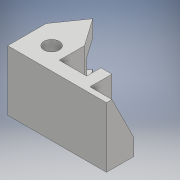
# Autodesk Inventor part: P4-10
Saved by Autodesk Inventor 2017 (Build 210142000, 142)
## iProperties
Created: 2017-03-01
Part Number: P4-10
Material: Generic
Document SubType Name: Modeling
Designer: Schaffel
Density: 1 g/cm^3
Appearance: Default
Author: Schaffel
Autodesk Inventor part; units mm, degrees
ref_plane "YZ Plane" through (0, 0, 0) normal (1, 0, 0) x (0, 1, 0)
ref_plane "XZ Plane" through (0, 0, 0) normal (0, 1, 0) x (-1, 0, 0)
ref_plane "XY Plane" through (0, 0, 0) normal (0, 0, 1) x (1, 0, 0)
sketch "Sketch1" plane through (0, 0, 0) normal (0, 0, 1) x (1, 0, 0)
  line L0 (0, 0) -> (90, 0)
  line L1 (90, 0) -> (90, 25)
  line L2 (90, 25) -> (60, 25)
  line L3 (60, 25) -> (60, 12)
  line L4 (60, 12) -> (35, 12)
  line L5 (35, 12) -> (35, 35)
  line L6 (0, 0) -> (0, 35)
  line L7 (17.5, 60) -> (0, 35)
  line L8 (17.5, 60) -> (35, 35)
  circle A0 centre (20, 20) radius 7
  dimension "d0" = 90
  dimension "d1" = 25
  constraints: 18 end point, 5 perpendicular, 1 centre point, 1 horizontal, 1 vertical
  measures "d0" distance of L0.start L0.end
  measures "d1" distance of L0.end L1.end
extrude "Extrusion1" add sketch "Sketch1" along normal blind 55
sketch "Sketch2" plane through (90, 0, 0) normal (1, 0, 0) x (0, 0, -1)
  line L0 (0, 25) -> (-55, 25) projected
  line L1 (-15, 25) -> (-55, 25)
  line L2 (-55, 35) -> (-55, 0) projected
  line L3 (-55, 5) -> (-15, 25)
  line L4 (-55, 25) -> (-55, 5)
  line L5 (-55, 12) -> (-55, 35) projected
  point P0 (0, 0)
  constraints: 6 end point, 3 point on line, 1 collinear, 1 horizontal
extrude "Extrusion2" cut sketch "Sketch2" against normal blind 20
sketch "Sketch3" plane through (35, 12, 0) normal (1, 0, 0) x (0, 0, -1)
  line L0 (0, 48) -> (-55, 48) projected
  line L1 (-15, 48) -> (-15, 30)
  line L2 (0, 23) -> (-55, 23) projected
  line L3 (-15, 30) -> (-40, 30)
  line L4 (-40, 30) -> (-40, 48)
  line L5 (-15, 48) -> (-40, 48)
  point P0 (0, -12)
  dimension "d6" = 18
  constraints: 8 end point, 3 perpendicular, 2 point on line, 1 horizontal
  measures "d6" distance of L1.start L1.end
extrude "Extrusion3" cut sketch "Sketch3" against normal blind 35
body "Solid1"
